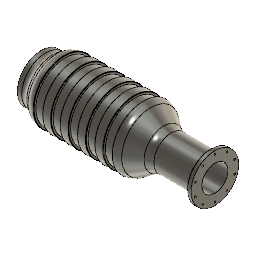
central_mounting_shaft_eng_model (Autodesk Fusion 360 design; units mm, degrees)
Autodesk Fusion 360 part; units mm, degrees
sketch "Sketch1" plane through (0, 0, 0) normal (0, 1, 0) x (1, 0, 0)
  line L0 (-0.0832, -72.005) -> (399.9168, -72.005) construction
  line L1 (399.9168, -72.005) -> (399.9168, 0) construction
  line L2 (399.9168, -30) -> (399.9168, -55)
  line L3 (399.9168, -55) -> (389.9168, -55)
  line L4 (389.9168, -55) -> (389.9168, -40)
  line L5 (389.9168, -40) -> (289.9168, -40)
  line L6 (-0.0767, -25) -> (-0.0767, -55)
  line L7 (-0.0767, -55) -> (19.9233, -55)
  line L8 (19.9233, -55) -> (44.2089, -72.005)
  line L9 (289.9168, -40) -> (244.2089, -72.005)
  line L10 (44.2089, -72.005) -> (244.2089, -72.005)
  line L11 (9.9233, -25) -> (9.9233, -45)
  line L12 (9.9233, -45) -> (23.0763, -45)
  line L13 (23.0763, -45) -> (47.3619, -62.005)
  line L14 (47.3619, -62.005) -> (241.0559, -62.005)
  line L15 (286.7638, -30) -> (241.0559, -62.005)
  line L16 (389.9168, -30) -> (286.7638, -30)
  line L17 (389.9168, -30) -> (399.9168, -30)
  line L18 (-0.0767, -25) -> (9.9233, -25)
  point P0 (399.9168, -30)
  dimension "d1" = 400
  dimension "d2" = 72.005
  dimension "d3" = 72.005
  dimension "d4" = 30
  dimension "d5" = 55
  dimension "d6" = 10
  dimension "d7" = 15
  dimension "d8" = 100
  dimension "d10" = 25
  dimension "d11" = 55
  dimension "d12" = 20
  dimension "d15" = 145
  dimension "d17" = 145
  dimension "d18" = 200
  dimension "d19" = -10
  constraint horizontal L0
  constraint perpendicular L0 L1
  constraint coincident L1 P0
  constraint coincident P0 L2.start
  constraint coincident L1 L2.end
  constraint perpendicular L1 L3
  constraint perpendicular L3 L4
  constraint perpendicular L4 L5
  constraint vertical L6
  constraint perpendicular L6 L7
  constraint coincident L0 L8.end
  constraint coincident L0 L9.end
  measures "d1" distance of L0.start L0.end
  measures "d2" distance of L0.end L1.end
  measures "d3" distance of origin L0
  measures "d4" distance of L1.end P0
  measures "d5" distance of L1.end L2.end
  measures "d6" distance of L2.end L3.end
  measures "d7" distance of L3.end L4.end
  measures "d8" distance of L4.end L5.end
  measures "d10" vertical distance of origin L6.start
  measures "d11" vertical distance of origin L6.end
  measures "d12" distance of L6.end L7.end
  measures "d15" angle of L7 L8
  measures "d17" angle of L5 L9
  measures "d18" distance of L8.end L9.end
revolve "Revolve1" add sketch "Sketch1" angle 360 about axis through (1.75, 0, 0) along (1, 0, 0)
sketch "Sketch2" plane through (0, 0, 0) normal (0, 1, 0) x (1, 0, 0)
  line L0 (244.2089, 72.005) -> (244.2089, -72.005)
  line L1 (44.2089, 72.005) -> (44.2089, -72.005)
  line L2 (-0.0767, 55) -> (-0.0767, -55)
  line L3 (399.9168, 55) -> (399.9168, -55)
  line L4 (389.9168, 55) -> (389.9168, 40)
  line L5 (389.9168, -40) -> (389.9168, -55)
  line L6 (399.9168, 55) -> (389.9168, 55)
  line L7 (399.9168, -55) -> (389.9168, -55)
  line L8 (389.9168, 40) -> (289.9168, 40)
  line L9 (389.9168, -40) -> (289.9168, -40)
  line L10 (289.9168, 40) -> (244.2089, 72.005)
  line L11 (289.9168, -40) -> (244.2089, -72.005)
  line L12 (244.2089, 72.005) -> (44.2089, 72.005)
  line L13 (244.2089, -72.005) -> (44.2089, -72.005)
  line L14 (19.9233, -55) -> (44.2089, -72.005)
  line L15 (19.9233, 55) -> (44.2089, 72.005)
  line L16 (19.9233, 55) -> (-0.0767, 55)
  line L17 (19.9233, -55) -> (-0.0767, -55)
  line L18 (54.9233, -72.005) -> (74.9233, -72.005)
  line L19 (74.9233, -72.005) -> (74.9233, -67.005)
  line L20 (74.9233, -67.005) -> (54.9233, -67.005)
  line L21 (54.9233, -67.005) -> (54.9233, -72.005)
  dimension "d21" = 5
  dimension "d22" = 20
  dimension "d23" = 55
  constraint horizontal L18
  constraint vertical L19
  constraint horizontal L20
  constraint vertical L21
  constraint coincident L13 L18.start
  measures "d21" distance of L18.end L19.end
  measures "d22" distance of L18.start L18.end
  measures "d23" distance of L2 L21
revolve "Revolve2" cut sketch "Sketch2" angle 360 about axis through (-0.0767, 0, 0) along (1, 0, 0) contours L13 L18 L19 L20 L21
pattern_linear "R-Pattern1" count 5 spacing 40 along (1, 0, 0) of "Revolve2"
fillet "Fillet1" radius 30 1 edges at (19.9233, -19.8888, -51.278)
fillet "Fillet1" radius 30 1 edges at (289.9168, -14.4646, -37.2931)
fillet "Fillet1" radius 30 1 edges at (244.2089, -26.0381, -67.1322)
fillet "Fillet1" radius 30 1 edges at (44.2089, -26.0381, -67.1322)
chamfer "Chamfer1" distance 1 angle 45 10 edges at (54.9233, -26.0381, -67.1322) (74.9233, 26.0381, -67.1322) (94.9233, 26.0381, -67.1322) (114.9233, -26.0381, -67.1322) (134.9233, 26.0381, -67.1322) (154.9233, -26.0381, -67.1322) (174.9233, 26.0381, -67.1322) (194.9233, -26.0381, -67.1322) (214.9233, 26.0381, -67.1322) (234.9233, -26.0381, -67.1322) measured on face at (54.0864, 7.1694, 71.6472) measured on face at (81.5899, 3.5892, 71.9155) measured on face at (94.9233, 3.5773, 70.0703) measured on face at (114.9233, 3.5773, 70.0703) measured on face at (134.9233, 3.5773, 70.0703) measured on face at (154.9233, 3.5773, 70.0703) measured on face at (174.9233, 3.5773, 70.0703) measured on face at (194.9233, 3.5773, 70.0703) measured on face at (214.9233, 3.5773, 70.0703) measured on face at (234.9233, -6.9061, 69.8205)
fillet "Fillet2" radius 2 1 edges at (389.9168, -14.4646, -37.2931)
chamfer "Chamfer2" distance 2 angle 45 1 edges at (389.9168, -19.8888, -51.278) measured on face at (389.9168, 4.819, 50.3055)
sketch "Sketch3" plane through (-0.0767, 0, 0) normal (-1, 0, 0) x (0, -1, 0)
  circle A0 centre (0, 0) radius 55
  circle A1 centre (0, 0) radius 25
  line L0 (0, 0) -> (-0.7815, 0) construction
  line L1 (0, 0) -> (0, 76.3803) construction
  circle A2 centre (0, 45) radius 2
  dimension "d43" = 4
  dimension "d44" = 45
  constraint coincident A0.centre A1.centre
  constraint horizontal L0
  constraint perpendicular L0 L1
  constraint coincident L1 A2.centre
  measures "d43" diameter of A2
  measures "d44" distance of A0.centre A2.centre
extrude "Extrude1" cut sketch "Sketch3" along normal mid plane 20 contours A2
pattern_circular "C-Pattern1" count 10 over 360 about axis through (1.75, 0, 0) along (1, 0, 0) of "Extrude1"
sketch "Sketch4" plane through (399.9168, 0, 0) normal (1, 0, 0) x (0, 1, 0)
  circle A0 centre (0, 0) radius 30
  circle A1 centre (0, 0) radius 55
  line L0 (0, 0) -> (0, 4.3991)
  line L1 (0, 4.3991) -> (0, 62.5149) construction
  circle A2 centre (0, 47.5) radius 2
  dimension "d49" = 4
  dimension "d50" = 47.5
  constraint coincident A0.centre A1.centre
  constraint vertical L0
  constraint parallel L0 L1
  constraint coincident L1 A2.centre
  measures "d49" diameter of A2
  measures "d50" distance of A0.centre A2.centre
extrude "Extrude2" cut sketch "Sketch4" along normal mid plane 40 contours A2
pattern_circular "C-Pattern2" count 10 over 360 about axis through (1.75, 0, 0) along (1, 0, 0) of "Extrude2"
equation "d2 = ( 144.01 / 2 ) * 1 mm"
